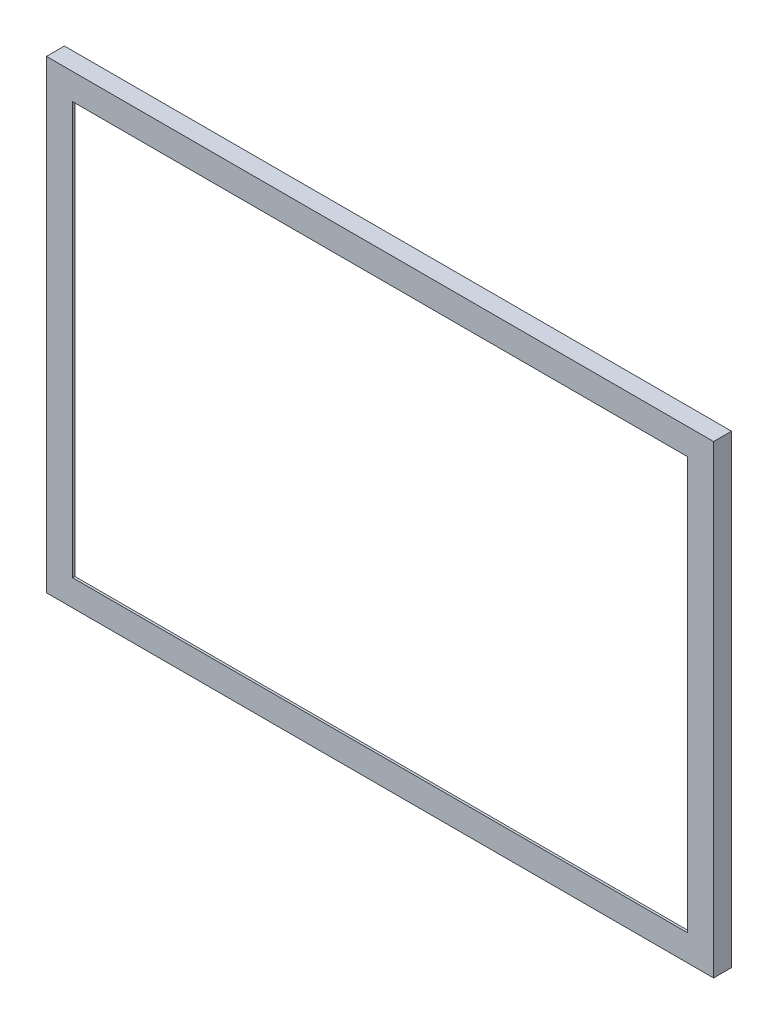
# Autodesk Inventor part: DummyAuschnitt
Saved by Autodesk Inventor 2017 (Build 210142000, 142)
## iProperties
Part Number: DummyAuschnitt
Material: Generisch
Document SubType Name: Modeling
Designer: aXe
Density: 1 g/cm^3
Appearance: Vorgabe
Author: aXe
Autodesk Inventor part; units mm, degrees
ref_plane "YZ Plane" through (0, 0, 0) normal (1, 0, 0) x (0, 1, 0)
ref_plane "XZ Plane" through (0, 0, 0) normal (0, 1, 0) x (-1, 0, 0)
ref_plane "XY Plane" through (0, 0, 0) normal (0, 0, 1) x (1, 0, 0)
ref_plane "Arbeitsebene1" through (0, 0, 0) normal (0, 0, 1) x (1, 0, 0)
sketch "Skizze1" plane through (0, 0, 0) normal (0, 0, 1) x (1, 0, 0)
  line L0 (47.05, -35.35) -> (47.05, 27.75) projected
  line L1 (47.05, 27.75) -> (-47.05, 27.75) projected
  line L2 (-47.05, 27.75) -> (-47.05, -35.35) projected
  line L3 (-47.05, -35.35) -> (47.05, -35.35) projected
  line L4 (-47.05, 27.75) -> (-47.15, 27.75)
  line L5 (-47.15, 27.75) -> (-47.15, 27.85)
  line L6 (-47.15, 27.85) -> (-47.05, 27.85)
  line L7 (-47.05, 27.85) -> (-47.05, 27.75)
  line L8 (47.05, -35.35) -> (47.15, -35.35)
  line L9 (47.15, -35.35) -> (47.15, -35.45)
  line L10 (47.15, -35.45) -> (47.05, -35.45)
  line L11 (47.05, -35.45) -> (47.05, -35.35)
  line L12 (-47.15, 27.85) -> (47.15, 27.85)
  line L13 (47.15, 27.85) -> (47.15, -35.45)
  line L14 (47.15, -35.45) -> (-47.15, -35.45)
  line L15 (-47.15, -35.45) -> (-47.15, 27.85)
  point P0 (0, 0)
  dimension "d0" = 0.1
  dimension "d1" = 0.1
  dimension "d2" = 0.1
  dimension "d3" = 0.1
  constraints: 24 end point, 6 parallel, 3 horizontal, 3 perpendicular
  measures "d0" distance of L5.end L6.end
  measures "d1" distance of L4.end L5.end
  measures "d2" distance of L9.end L10.end
  measures "d3" distance of L8.end L9.end
ref_plane "Arbeitsebene2" through (-47.05, -35.35, -2.75) normal (0, 0, -1) x (0, 1, 0)
ref_plane "Arbeitsebene3" through (0, 0, 0) normal (0, 0, 1) x (1, 0, 0)
ref_plane "Arbeitsebene4" through (-47.05, -35.35, -2.75) normal (0, 0, -1) x (0, 1, 0)
sketch "Skizze2" plane through (0, 0, 0) normal (0, 0, 1) x (1, 0, 0)
  line L0 (47.05, -35.35) -> (47.05, 27.75) projected
  line L1 (47.05, 27.75) -> (-47.05, 27.75) projected
  line L2 (-47.05, 27.75) -> (-47.05, -35.35) projected
  line L3 (-47.05, -35.35) -> (47.05, -35.35) projected
  line L4 (-47.05, 27.75) -> (-51.05, 27.75)
  line L5 (-51.05, 27.75) -> (-51.05, 31.75)
  line L6 (-51.05, 31.75) -> (-47.05, 31.75)
  line L7 (-47.05, 31.75) -> (-47.05, 27.75)
  line L8 (47.05, -35.35) -> (51.05, -35.35)
  line L9 (51.05, -35.35) -> (51.05, -39.35)
  line L10 (51.05, -39.35) -> (47.05, -39.35)
  line L11 (47.05, -39.35) -> (47.05, -35.35)
  line L12 (-51.05, 31.75) -> (51.05, 31.75)
  line L13 (51.05, 31.75) -> (51.05, -39.35)
  line L14 (51.05, -39.35) -> (-51.05, -39.35)
  line L15 (-51.05, -39.35) -> (-51.05, 31.75)
  point P0 (0, 0)
  dimension "d6" = 4
  dimension "d7" = 4
  dimension "d8" = 4
  dimension "d9" = 4
  constraints: 24 end point, 6 parallel, 3 horizontal, 3 perpendicular
  measures "d6" distance of L5.end L6.end
  measures "d7" distance of L4.end L5.end
  measures "d8" distance of L9.end L10.end
  measures "d9" distance of L8.end L9.end
extrude "Extrusion2" add sketch "Skizze2" against normal up to surface (2.75 mm away)
extrude "Extrusion3" cut sketch "Skizze1" against normal up to surface (2.75 mm away) contours L3 L2 L1 L0
chamfer "Fase1" distance 2.4 angle 45 4 edges at (0, -35.35, -2.75) (-47.05, -3.8, -2.75) (47.05, -3.8, -2.75) (0, 27.75, -2.75)
